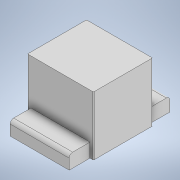
# Autodesk Inventor part: base_of_linear_motor
Saved by Autodesk Inventor 2022 (Build 260153000, 153)
## iProperties
Created: 2022-08-25
Part Number: base_of_linear_motor
Material: Generic
Document SubType Name: Modeling
Designer: Alok
Density: 1 g/cm^3
Appearance: Default
Author: Alok
Autodesk Inventor part; units mm, degrees
ref_plane "YZ Plane" through (0, 0, 0) normal (1, 0, 0) x (0, 1, 0)
ref_plane "XZ Plane" through (0, 0, 0) normal (0, 1, 0) x (-1, 0, 0)
ref_plane "XY Plane" through (0, 0, 0) normal (0, 0, 1) x (1, 0, 0)
sketch "Sketch1" plane through (0, 0, 0) normal (0, 1, 0) x (-1, 0, 0)
  line L0 (47.5, 42.5) -> (-47.5, 42.5)
  line L1 (-47.5, 42.5) -> (-47.5, -42.5)
  line L2 (-47.5, -42.5) -> (47.5, -42.5)
  line L3 (47.5, -42.5) -> (47.5, 42.5)
  line L4 (47.5, 42.5) -> (-47.5, -42.5) construction
  line L5 (-47.5, 42.5) -> (47.5, -42.5) construction
  point P0 (0, 0)
  dimension "d0" = 95
  dimension "d1" = 85
  constraints: 12 end point, 2 midpoint, 2 parallel, 1 horizontal, 1 perpendicular
  measures "d0" distance of L1.end L2.end
  measures "d1" distance of L0.end L1.end
extrude "Extrusion1" add sketch "Sketch1" along normal blind 85
fillet "Face Fillet1" radius 1 1 edges at (47.5, 42.5, 42.5)
fillet "Face Fillet2" radius 1 1 edges at (47.5, 42.5, -42.5)
fillet "Face Fillet3" radius 1 1 edges at (-47.5, 42.5, -42.5)
fillet "Face Fillet4" radius 1 1 edges at (-47.5, 42.5, 42.5)
sketch "Sketch2" plane through (46.5, 0, -42.5) normal (0, 0, -1) x (-1, 0, 0)
  line L0 (89, 0) -> (89, 20)
  line L1 (89, 20) -> (4, 20)
  line L2 (4, 20) -> (4, 0)
  line L3 (89, 0) -> (4, 0)
  point P0 (46.5, 0)
  point P1 (94, 0)
  dimension "d9" = 20
  dimension "d10" = 85
  constraints: 8 end point, 2 perpendicular
  measures "d9" distance of L0.start L0.end
  measures "d10" distance of L0.end L1.end
extrude "Extrusion2" add sketch "Sketch2" along normal blind 30
mirror "Mirror1" about plane through (0, 0, 0) normal (0, 0, 1) of "Extrusion2"
fillet "Face Fillet5" radius 5 1 edges at (0, 20, 72.5)
fillet "Face Fillet6" radius 5 1 edges at (0, 20, -72.5)
sketch "Sketch3" plane through (-47.5, 0, -41.5) normal (-1, 0, 0) x (0, 0, 1)
  point P0 (41.5, 0)
body "Solid1"
